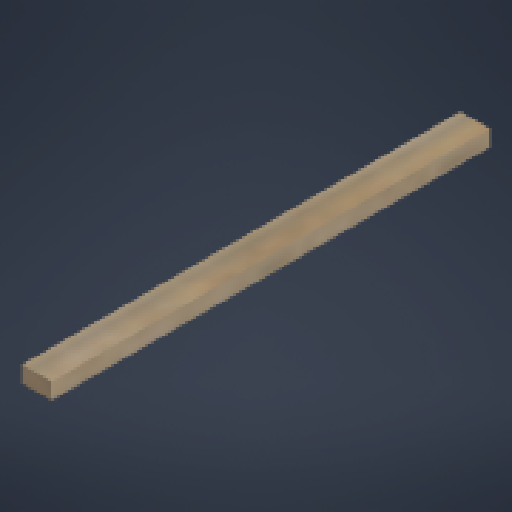
# Autodesk Inventor part: back_upper
Saved by Autodesk Inventor 2026.1 (Build 301233020, 233B)
## iProperties
Created: 2025-09-28
Part Number: back_upper
Material: 木材 (カエデ材)
Document SubType Name: Modeling
Designer: hibik
Density: 0.67 g/cm^3
Appearance: ナチュラル カエデ材 - 光沢 濃い着色
Author: hibik
Autodesk Inventor part; units mm, degrees
ref_plane "YZ Plane" through (0, 0, 0) normal (1, 0, 0) x (0, 1, 0)
ref_plane "XZ Plane" through (0, 0, 0) normal (0, 1, 0) x (-1, 0, 0)
ref_plane "XY Plane" through (0, 0, 0) normal (0, 0, 1) x (1, 0, 0)
sketch "スケッチ1" plane through (0, 0, 0) normal (0, 1, 0) x (-1, 0, 0)
  line L0 (0, 99) -> (10, 99)
  line L1 (10, 99) -> (10, -99)
  line L2 (10, -99) -> (0, -99)
  line L3 (0, -99) -> (0, 99)
  point P0 (0, 0)
  point P1 (0, 0)
  dimension "d0" = 198
  dimension "d1" = 10
  constraints: 8 end point, 2 parallel, 1 coincident, 1 horizontal, 1 midpoint, 1 perpendicular
  measures "d0" distance of L0.end L1.end
  measures "d1" distance of L0.start L0.end
extrude "押し出し1" add sketch "スケッチ1" along normal blind 5.5
sketch "スケッチ2" plane through (0, 5.5, 0) normal (0, 1, 0) x (1, 0, 0)
  line L0 (-10, 99) -> (-10, -99) projected
  line L1 (-10, -99) -> (0, -99)
  line L2 (0, -99) -> (0, -74)
  line L3 (0, -74) -> (-10, -74)
  line L4 (-10, -74) -> (-10, -99)
  line L5 (0, -99) -> (0, 98.6733)
  point P0 (0, 0)
  point P1 (-10, -74)
  dimension "d4" = 25
  dimension "d7" = 10
  constraints: 10 end point, 2 parallel, 1 collinear, 1 horizontal, 1 perpendicular
  measures "d4" distance of L1.end L2.end
  measures "d7" distance of L0.end L1.end
extrude "押し出し2" cut sketch "スケッチ2" against normal through all
mirror "ミラー1" about plane through (0, 0, 0) normal (0, 0, 1) of "押し出し2"
